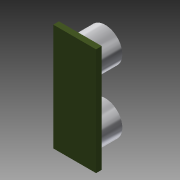
# Autodesk Inventor part: Sonar
Saved by Autodesk Inventor 2015 (Build 190159000, 159)
## iProperties
Created: 2016-11-29
Part Number: Sonar
Material: Generic
Document SubType Name: Modeling
Designer: James Yelland
Density: 1 g/cm^3
Appearance: Default
Author: James Yelland
Autodesk Inventor part; units mm, degrees
ref_plane "YZ Plane" through (0, 0, 0) normal (1, 0, 0) x (0, 1, 0)
ref_plane "XZ Plane" through (0, 0, 0) normal (0, 1, 0) x (-1, 0, 0)
ref_plane "XY Plane" through (0, 0, 0) normal (0, 0, 1) x (1, 0, 0)
sketch "Sketch1" plane through (0, 0, 0) normal (0, 1, 0) x (-1, 0, 0)
  line L0 (-6, -15) -> (-6, 15)
  line L1 (-6, 15) -> (6, 15)
  line L2 (6, 15) -> (6, -15)
  line L3 (6, -15) -> (-6, -15)
  line L4 (-6, -15) -> (6, 15) construction
  line L5 (-6, 15) -> (6, -15) construction
  line L6 (-6, -15) -> (24, -15) construction
  point P0 (0, 0)
  dimension "d0" = 30
  dimension "d1" = 90
  dimension "d2" = 12
  constraints: 14 end point, 2 midpoint, 2 parallel, 2 perpendicular, 1 horizontal, 1 vertical
  measures "d0" distance of L0.start L0.end
  measures "d1" angle of L6 L0
  measures "d2" distance of L0.end L1.end
extrude "Extrusion1" add sketch "Sketch1" along normal blind 1.6
sketch "Sketch2" plane through (0, 1.6, 0) normal (0, 1, 0) x (1, 0, 0)
  line L0 (0, 0) -> (0, -8.89)
  line L1 (0, 0) -> (8.89, 0) construction
  line L2 (0, -8.89) -> (0, 8.89)
  circle A0 centre (0, -8.89) radius 4.75
  circle A1 centre (0, 8.89) radius 4.75
  dimension "d5" = 8.89
  dimension "d6" = 90
  dimension "d7" = 17.78
  dimension "d8" = 0
  dimension "d9" = 9.5
  dimension "d10" = 9.5
  constraints: 6 end point, 2 centre point, 2 coincident, 1 collinear, 1 horizontal, 1 perpendicular, 1 vertical
  measures "d5" distance of L0.start L0.end
  measures "d6" angle of L0 L1
  measures "d7" distance of L0.end L2.end
  measures "d8" distance between parallel lines of L2 L0
  measures "d9" diameter of A0
  measures "d10" diameter of A1
extrude "Extrusion2" add sketch "Sketch2" along normal blind 7
sketch "Sketch3" plane through (0, 8.6, 8.89) normal (0, 1, 0) x (1, 0, 0)
  circle A0 centre (0, 0) radius 3.5
  line L0 (0, 8.89) -> (0, 17.78)
  circle A1 centre (0, 17.78) radius 3.5
  dimension "d13" = 7
  dimension "d14" = 8.89
  dimension "d15" = 7
  constraints: 2 centre point, 2 end point, 1 coincident, 1 vertical
  measures "d13" diameter of A0
  measures "d14" distance of L0.start L0.end
  measures "d15" diameter of A1
extrude "Extrusion3" cut sketch "Sketch3" against normal blind 1
body "Solid1"
